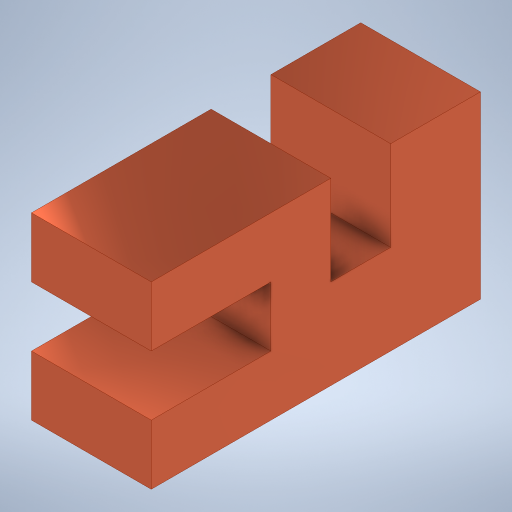
# Autodesk Inventor part: desenho 2,
Saved by Autodesk Inventor 2024 (Build 280153000, 153)
## iProperties
Created: 2023-09-11
Part Number: desenho 2,
Material: Generic
Document SubType Name: Modeling
Designer: LORAC
Density: 1 g/cm^3
Appearance: Metal 1400F Hot
Author: LORAC
Autodesk Inventor part; units mm, degrees
ref_plane "YZ Plane" through (0, 0, 0) normal (1, 0, 0) x (0, 1, 0)
ref_plane "XZ Plane" through (0, 0, 0) normal (0, 1, 0) x (-1, 0, 0)
ref_plane "XY Plane" through (0, 0, 0) normal (0, 0, 1) x (1, 0, 0)
sketch "Sketch1" plane through (0, 0, 0) normal (1, 0, 0) x (0, 1, 0)
  line L0 (0, 0) -> (0, -55)
  line L1 (0, -55) -> (30, -55)
  line L2 (30, -55) -> (30, -40)
  line L3 (30, -40) -> (15, -40)
  line L4 (15, -40) -> (15, -30)
  line L5 (15, -30) -> (30, -30)
  line L6 (30, -30) -> (30, 0)
  line L7 (30, 0) -> (20, 0)
  line L8 (20, 0) -> (20, -20)
  line L9 (20, -20) -> (10, -20)
  line L10 (10, -20) -> (10, 0)
  line L11 (10, 0) -> (0, 0)
  dimension "d0" = 55
  dimension "d1" = 30
  dimension "d2" = 15
  dimension "d3" = 15
  dimension "d4" = 10
  dimension "d5" = 15
  dimension "d6" = 30
  dimension "d7" = 10
  dimension "d8" = 20
  dimension "d9" = 10
  constraints: 24 end point, 6 vertical, 5 horizontal, 1 perpendicular
  measures "d0" distance of L0.start L0.end
  measures "d1" distance of L0.end L1.end
  measures "d2" distance of L1.end L2.end
  measures "d3" distance of L2.end L3.end
  measures "d4" distance of L3.end L4.end
  measures "d5" distance of L4.end L5.end
  measures "d6" distance of L5.end L6.end
  measures "d7" distance of L6.end L7.end
  measures "d8" distance of L7.end L8.end
  measures "d9" distance of L8.end L9.end
extrude "Extrusion1" add sketch "Sketch1" along normal mid plane 20
body "Solid1"
